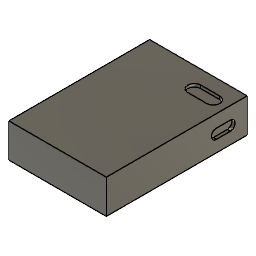
Behuizing4Volledig (Autodesk Fusion 360 archive; units mm, degrees)
design "PowerBankSizeUp"
part number: 2026-03-20-14-54-00-920
Autodesk Fusion 360 part; units mm, degrees
sketch "Sketch1" plane through (0, 0, 0) normal (0, 0, 1) x (1, 0, 0)
  line L0 (0, 0) -> (63, 0)
  line L1 (63, 0) -> (63, 91)
  line L2 (63, 91) -> (0, 91)
  line L3 (0, 91) -> (0, 0)
  dimension "d1" = 63
  dimension "d2" = 91
  constraint horizontal L0
  constraint vertical L1
  constraint horizontal L2
  constraint vertical L3
  constraint coincident L0.start L3.end
  measures "d1" distance of L1 L3
  measures "d2" distance of L0 L2
extrude "Extrude1" add sketch "Sketch1" along normal blind 22
sketch "Sketch2" plane through (0, 0, 22) normal (0, 0, 1) x (-1, 0, 0)
  line L0 (0, -91) -> (0, 0)
  line L1 (0, 0) -> (-63, 0)
  line L2 (-63, 0) -> (-63, -91)
  line L3 (-63, -91) -> (0, -91)
  line L4 (-42, -82.0063) -> (-54.229, -82.0063)
  arc A0 (-54.229, -73.6334) -> (-54.229, -82.0063) centre (-54.229, -77.8199) ccw
  line L5 (-54.229, -73.6334) -> (-42, -73.6334)
  arc A1 (-42, -82.0063) -> (-42, -73.6334) centre (-42, -77.8199) ccw
  dimension "d9" = 42
  dimension "d10" = 8.771
  constraint horizontal L4
  constraint tangent L4 A0
  constraint tangent A0 L5
  constraint parallel L4 L5
  constraint tangent L5 A1
  constraint tangent L4 A1
  measures "d9" distance of L0 A1.centre
  measures "d10" distance of L2 A0.centre
extrude "Extrude2" cut sketch "Sketch2" against normal blind 2 contours L4 A0 L5 A1
sketch "Sketch3" plane through (63, 0, 0) normal (1, 0, 0) x (0, 1, 0)
  line L0 (0, 0) -> (91, 0)
  line L1 (91, 0) -> (91, 22)
  line L2 (91, 22) -> (0, 22)
  line L3 (0, 22) -> (0, 0)
  line L4 (71, 13.87) -> (80, 13.87)
  arc A0 (80, 7.6199) -> (80, 13.87) centre (80, 10.7449) ccw
  line L5 (80, 7.6199) -> (71, 7.6199)
  arc A1 (71, 13.87) -> (71, 7.6199) centre (71, 10.7449) ccw
  dimension "d11" = 8.13
  constraint horizontal L4
  constraint tangent L4 A0
  constraint tangent A0 L5
  constraint parallel L4 L5
  constraint tangent L5 A1
  constraint tangent L4 A1
  measures "d11" distance of L2 L4
extrude "Extrude3" cut sketch "Sketch3" against normal blind 2 contours L4 A0 L5 A1
move_body "Move2" bodies 1 to x (-1, 0, 0) y (0, 1, 0) z (0, 0, -1) at (63, 0, 22)
move_body "Move3" bodies 1 to x (-1, 0, 0) y (0, 1, 0) z (0, 0, -1) at (63, 0, 22)

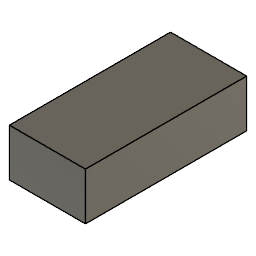
design "ESP32Afmetingen"
part number: 2026-03-19-13-57-27-742
Autodesk Fusion 360 part; units mm, degrees
sketch "Sketch1" plane through (0, 0, 0) normal (0, 0, 1) x (1, 0, 0)
  line L0 (0, 0) -> (25.57, 0)
  line L1 (25.57, 0) -> (25.57, 54.14)
  line L2 (25.57, 54.14) -> (0, 54.14)
  line L3 (0, 54.14) -> (0, 0)
  dimension "d1" = 54.14
  dimension "d2" = 25.57
  constraint horizontal L0
  constraint vertical L1
  constraint horizontal L2
  constraint vertical L3
  constraint coincident L0.start L3.end
  measures "d1" distance of L0.start L2.end
  measures "d2" distance of L1.end L2.end
extrude "Extrude1" add sketch "Sketch1" along normal blind 15.94
sketch "Sketch2" plane through (0, 54.14, 0) normal (0, 1, 0) x (-1, 0, 0)
  line L0 (-25.57, 0) -> (0, 0)
  line L1 (0, 0) -> (0, 15.94)
  line L2 (0, 15.94) -> (-25.57, 15.94)
  line L3 (-25.57, 15.94) -> (-25.57, 0)
  line L4 (-22.5, 10) -> (-17.5, 10)
  line L5 (-17.5, 10) -> (-17.5, 7.5)
  line L6 (-17.5, 7.5) -> (-22.5, 7.5)
  line L7 (-22.5, 7.5) -> (-22.5, 10)
  line L8 (-7.5, 10) -> (-2.5, 10)
  line L9 (-2.5, 10) -> (-2.5, 7.5)
  line L10 (-2.5, 7.5) -> (-7.5, 7.5)
  line L11 (-7.5, 7.5) -> (-7.5, 10)
  constraint horizontal L4
  constraint vertical L5
  constraint horizontal L6
  constraint vertical L7
  constraint horizontal L8
  constraint vertical L9
  constraint horizontal L10
  constraint vertical L11
extrude "Extrude2" cut sketch "Sketch2" against normal blind 1 contours L4 L5 L6 L7 | L8 L9 L10 L11
move_body "Move1" bodies 1 to x (1, 0, 0) y (0, 1, 0) z (0, 0, 1) at (19.6481, 55.9741, 0)
move_body "Move2" bodies 1 to x (1, 0, 0) y (0, 1, 0) z (0, 0, 1) at (0, -47, 0)
